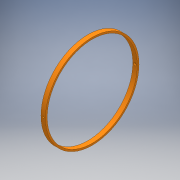
# Autodesk Inventor part: Outer Ring
Saved by Autodesk Inventor 2018 (Build 220112000, 112)
## iProperties
Created: 2018-03-07
Part Number: Outer Ring
Material: Generic
Document SubType Name: Modeling
Designer: sterl
Density: 1 g/cm^3
Appearance: Orange
Author: sterl
Autodesk Inventor part; units mm, degrees
ref_plane "YZ Plane" through (0, 0, 0) normal (1, 0, 0) x (0, 1, 0)
ref_plane "XY Plane" through (0, 0, 0) normal (0, 0, 1) x (1, 0, 0)
sketch "Sketch1" plane through (0, 0, 0) normal (1, 0, 0) x (0, 1, 0)
  circle A0 centre (0, 0) radius 106
  circle A1 centre (0, 0) radius 102
  dimension "d0" = 212
  dimension "d1" = 204
  constraints: 2 centre point, 2 coincident
  measures "d0" diameter of A0
  measures "d1" diameter of A1
extrude "Extrusion1" add sketch "Sketch1" along normal blind 10
ref_plane "Work Plane1" through (0, 106, 0) normal (0, 1, 0) x (-1, 0, 0)
sketch "Sketch2" plane through (0, 106, 0) normal (0, 1, 0) x (-1, 0, 0)
  line L0 (-10, 106) -> (-10, -106) projected
  line L1 (0, -106) -> (0, 106) projected
  line L2 (0, 0) -> (-10, 0)
  circle A0 centre (-5, 0) radius 2
  dimension "d4" = 4
  constraints: 2 end point, 2 midpoint, 1 centre point
  measures "d4" diameter of A0
extrude "Extrusion2" cut sketch "Sketch2" against normal blind 227.25
ref_plane "Work Plane2" through (0, 102, 0) normal (0, 1, 0) x (-1, 0, 0)
sketch "Sketch3" plane through (0, 102, 0) normal (0, 1, 0) x (-1, 0, 0)
  spline S0 degree 8 poles (-3, 0) (-3, 0.2418) (-3.0334, 0.4777) (-3.0974, 0.7026) (-3.1883, 0.9122) (-3.3019, 1.1027) (-3.4331, 1.2718) (-3.5763, 1.4179) (-3.8674, 1.6587) (-4.0179, 1.758) (-4.1746, 1.8396) (-4.3357, 1.9041) (-4.4998, 1.9522) (-4.6659, 1.984) (-4.8329, 2) (-5.1671, 2) (-5.3341, 1.984) (-5.5002, 1.9522) (-5.6643, 1.9041) (-5.8254, 1.8396) (-5.9821, 1.758) (-6.1326, 1.6587) (-6.3952, 1.4415) (-6.5105, 1.328) (-6.6186, 1.2004) (-6.7168, 1.059) (-6.8029, 0.9046) (-6.8744, 0.738) (-6.9291, 0.5608) (-7.0023, 0.1769) (-7.0176, -0.027) (-7.0089, -0.2323) (-6.9761, -0.4342) (-6.9207, -0.6282) (-6.8456, -0.8099) (-6.7549, -0.976) (-6.5833, -1.2285) (-6.5064, -1.3254) (-6.4246, -1.4147) (-6.3385, -1.4967) (-6.2487, -1.5713) (-6.156, -1.6388) (-6.0608, -1.6991) (-5.7701, -1.8589) (-5.5684, -1.9381) (-5.3616, -1.9912) (-5.1519, -2.0192) (-4.9413, -2.0224) (-4.7315, -2.001) (-4.5245, -1.9545) (-4.0782, -1.7938) (-3.8331, -1.6646) (-3.5983, -1.49) (-3.3853, -1.269) (-3.2062, -1.0033) (-3.0735, -0.6973) (-3, -0.3585) (-3, 0) knots 0 0 0 0 0 0 0 0 0 0.127516 0.127516 0.127516 0.127516 0.127516 0.127516 0.127516 0.249326 0.249326 0.249326 0.249326 0.249326 0.249326 0.249326 0.37114 0.37114 0.37114 0.37114 0.37114 0.37114 0.37114 0.474202 0.474202 0.474202 0.474202 0.474202 0.474202 0.474202 0.583798 0.583798 0.583798 0.583798 0.583798 0.583798 0.583798 0.660966 0.660966 0.660966 0.660966 0.660966 0.660966 0.660966 0.814386 0.814386 0.814386 0.814386 0.814386 0.814386 0.814386 1 1 1 1 1 1 1 1 1 projected
  line L0 (-7, 0) -> (-3, 0)
  circle A0 centre (-5, 0) radius 3
  point P0 (0, 0)
  dimension "d7" = 6
  constraints: 2 end point, 1 centre point, 1 horizontal, 1 midpoint, 3 other
  measures "d7" diameter of A0
extrude "Extrusion3" cut sketch "Sketch3" along normal mid plane 5
mirror "Mirror1" about plane through (0, 0, 0) normal (0, 1, 0) of "Extrusion3"
body "Solid1"
